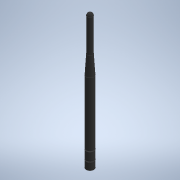
# Autodesk Inventor part: 900MHz_duck
Saved by Autodesk Inventor 2020.2 (Build 242310000, 310)
## iProperties
Created: 2020-04-11
Part Number: 900MHz_duck
Material: Rubber, Silicone
Document SubType Name: Modeling
Designer: agmlego
Mass: 12.5478 g
Surface Area: 48.859 cm^2
Volume: 10.0382 cm^3
Density: 1.25 g/cm^3
Appearance: Rubber - Black
Author: agmlego
Autodesk Inventor part; units mm, degrees
ref_plane "YZ Plane" through (0, 0, 0) normal (1, 0, 0) x (0, 1, 0)
ref_plane "XZ Plane" through (0, 0, 0) normal (0, 1, 0) x (-1, 0, 0)
ref_plane "XY Plane" through (0, 0, 0) normal (0, 0, 1) x (1, 0, 0)
sketch "Sketch1" plane through (0, 0, 0) normal (0, 0, 1) x (1, 0, 0)
  line L0 (0, 0) -> (0, 169.6466)
  arc A0 (3.41, 166.2367) -> (0, 169.6466) centre (0, 166.2367) ccw
  line L1 (3.41, 166.2367) -> (3.41, 124.6124)
  line L2 (3.41, 124.6124) -> (4.8069, 101.346)
  line L3 (4.8069, 101.346) -> (4.807, 83.3535)
  line L4 (4.807, 83.3535) -> (4.8069, 21.2471)
  line L5 (4.8069, 21.2471) -> (4.6355, 20.8661)
  line L6 (4.6355, 20.8661) -> (4.8069, 20.4851)
  line L7 (4.8069, 20.4851) -> (4.8069, 9.7409)
  line L8 (4.8069, 9.7409) -> (2.54, 9.7409)
  line L9 (2.54, 9.7409) -> (2.54, 9.2329)
  line L10 (2.54, 9.2329) -> (4.8069, 9.2329)
  line L11 (4.8069, 9.2329) -> (4.8069, 0)
  line L12 (4.8069, 0) -> (0, 0)
  dimension "d0" = 3.4099
  dimension "d1" = 4.8069
  dimension "d2" = 4.6355
  dimension "d3" = 0.762
  dimension "d4" = 2.54
  dimension "d5" = 0.508
  dimension "d6" = 9.2329
  dimension "d7" = 10.7442
  dimension "d8" = 80.0989
  dimension "d9" = 23.2664
  dimension "d10" = 45.0342
  dimension "d11" = 169.6466
  constraints: 26 end point, 5 point on line, 4 perpendicular, 2 parallel, 2 point on circle, 2 vertical, 1 centre point, 1 collinear, 1 equal length, 1 line through centre, 1 tangent
  measures "d0" distance between parallel lines of L0 L1
  measures "d1" distance between parallel lines of L0 L3
  measures "d2" distance from line of L0 L5.end
  measures "d3" distance of L6.end L4.end
  measures "d4" distance between parallel lines of L0 L9
  measures "d5" distance of L8.end L9.end
  measures "d6" distance of L10.end L11.end
  measures "d7" distance of L6.end L7.end
  measures "d8" distance of L4.end L2.end
  measures "d9" vertical distance of L2.end L1.end
  measures "d10" vertical distance of L0.end L1.end
  measures "d11" distance of L0.start L0.end
revolve "Revolution1" add sketch "Sketch1" angle 360 about axis through (0, 0, 0) along (0, 1, 0)
sketch "Sketch2" plane through (0, 0, 0) normal (0, -1, 0) x (1, 0, 0)
  circle A0 centre (0, 0) radius 4.8069 projected
  constraints: 1 coincident
hole "Hole1" at (0, 0, 0) direction (0, 1, 0) diameter 5.588 depth 5.6261 thread size "1/4-36 UNS" class "2B" standard "ANSI Unified Screw Threads"
fillet "Fillet1" radius 0.25 9 edges at (-4.8069, 9.2329, 0) (-4.8069, 0, 0) (-4.8069, 9.7409, 0) (0, 0, 2.794) (-4.8069, 20.4851, 0) (-4.6355, 20.8661, 0) (-4.8069, 21.2471, 0) (-4.8069, 101.346, 0) (-3.41, 124.6124, 0)
body "Solid1"
